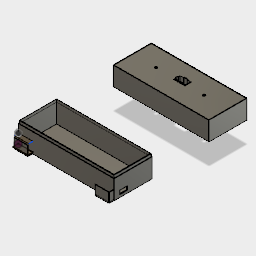
Breadboard case v11 (Autodesk Fusion 360 design; units mm, degrees)
Autodesk Fusion 360 part; units mm, degrees
sketch "Sketch1" plane through (0, 0, 0) normal (0, 1, 0) x (1, 0, 0)
  line L0 (100, 40) -> (-100, 40)
  line L1 (-100, 40) -> (-100, -40)
  line L2 (-100, -40) -> (100, -40)
  line L3 (100, -40) -> (100, 40)
  line L4 (100, 40) -> (-100, -40) construction
  line L5 (-100, 40) -> (100, -40) construction
  line L6 (-99, -39) -> (99, -39)
  line L7 (99, -39) -> (99, 39)
  line L8 (99, 39) -> (-99, 39)
  line L9 (-99, 39) -> (-99, -39)
  dimension "d1" = 200
  dimension "d2" = 80
  dimension "d3" = 1
  measures "d1" distance of L1.end L2.end
  measures "d2" distance of L0.end L1.end
extrude "Extrude1" add sketch "Sketch1" along normal blind 80 contours L0 L1 L2 L3 | L6 L7 L8 L9 makes body 1
shell "Shell1" thickness 1 removed faces 0 bodies 1
ref_plane "WorkPlane1" through (0, 40, 0) normal (0, 1, 0) x (0, 0, 1)
split "Split1" by plane through (0, 40, 0) normal (0, 1, 0) bodies 1 makes body 2 at (-33.3333, 80, -13.3333)
move_body "Move1" bodies 1 to x (1, 0, 0) y (0, 1, 0) z (0, 0, 1) at (-36.228, -3.4098, 161.9901)
sketch "Sketch2" plane through (0, -2.4098, 0) normal (0, 1, 0) x (-1, 0, 0)
  line L0 (-62.772, 200.9901) -> (-62.772, 122.9901)
  line L1 (-62.772, 122.9901) -> (135.228, 122.9901)
  line L2 (135.228, 122.9901) -> (135.228, 200.9901)
  line L3 (135.228, 200.9901) -> (-62.772, 200.9901)
  line L4 (135.228, 200.9901) -> (-62.772, 200.9901)
  line L5 (-62.772, 200.9901) -> (-62.772, 122.9901)
  line L6 (-62.772, 122.9901) -> (135.228, 122.9901)
  line L7 (135.228, 122.9901) -> (135.228, 200.9901)
  line L8 (-63.772, 121.9901) -> (136.228, 121.9901)
  line L9 (136.228, 121.9901) -> (136.228, 201.9901)
  line L10 (136.228, 201.9901) -> (-63.772, 201.9901)
  line L11 (-63.772, 201.9901) -> (-63.772, 121.9901)
  line L12 (135.228, 122.9901) -> (-62.772, 122.9901)
  line L13 (-62.772, 122.9901) -> (-62.772, 200.9901)
  line L14 (-62.772, 200.9901) -> (135.228, 200.9901)
  line L15 (135.228, 200.9901) -> (135.228, 122.9901)
  line L16 (-61.772, 199.9901) -> (-61.772, 123.9901)
  line L17 (-61.772, 123.9901) -> (134.228, 123.9901)
  line L18 (134.228, 123.9901) -> (134.228, 199.9901)
  line L19 (134.228, 199.9901) -> (-61.772, 199.9901)
  dimension "d7" = 1
  dimension "d8" = 1
extrude "Extrude2" add sketch "Sketch2" along normal blind 45 contours L0 L1 L2 L3 L4 L5 L6 L7 L12 L13 L14 L15 bodies 1
sketch "Sketch3" plane through (63.772, 0, 0) normal (1, 0, 0) x (0, 0, -1)
  line L0 (-121.9901, 36.5902) -> (-201.9901, 36.5902)
  line L1 (-201.9901, 36.5902) -> (-201.9901, -3.4098)
  line L2 (-201.9901, -3.4098) -> (-121.9901, -3.4098)
  line L3 (-121.9901, -3.4098) -> (-121.9901, 36.5902)
  line L4 (-190, 10) -> (-174, 10)
  line L5 (-174, 10) -> (-174, 2)
  line L6 (-174, 2) -> (-190, 2)
  line L7 (-190, 2) -> (-190, 10)
  dimension "d11" = 16
  dimension "d12" = 8
  measures "d11" distance of L4.start L4.end
  measures "d12" distance of L4.start L6.end
extrude "Extrude3" cut sketch "Sketch3" against normal up to surface (2 mm away) contours L4 L5 L6 L7 bodies 1
fillet "Fillet1" radius 0.5 4 edges at (-136.228, 16.5902, 121.9901) (-136.228, 16.5902, 201.9901) (63.772, 16.5902, 201.9901) (63.772, 16.5902, 121.9901) on bodies 1
chamfer "Chamfer1" distance 0.5 angle 45 4 edges at (-36.228, 42.5902, 200.9901) (62.772, 42.5902, 161.9901) (-36.228, 42.5902, 122.9901) (-135.228, 42.5902, 161.9901) on bodies 1
fillet "Fillet2" radius 0.5 9 edges at (0, 80, 40) (100, 80, 0) (100, 60, 40) (100, 60, -40) (0, 80, -40) (0, 40, -40) (-100, 80, 0) (-100, 40, 0) (0, 40, 40) on bodies 2
fillet "Fillet3" radius 0.5 9 edges at (-99.8536, 40.1464, -39.8536) (-100, 60, -40) (-99.8536, 79.8536, -39.8536) (-99.8536, 40.1464, 39.8536) (-100, 60, 40) (-99.8536, 79.8536, 39.8536) (-99, 79, 0) (0, 79, -39) (0, 79, 39) on bodies 2
sketch "Sketch4" plane through (0, 0, 121.9901) normal (0, 0, -1) x (-1, 0, 0)
  line L0 (-63.272, 36.5902) -> (-63.272, -3.4098)
  line L1 (-63.272, -3.4098) -> (135.728, -3.4098)
  line L2 (135.728, -3.4098) -> (135.728, 36.5902)
  line L3 (135.728, 36.5902) -> (-63.272, 36.5902)
  line L4 (-56, 18) -> (-40, 18)
  line L5 (-40, 18) -> (-40, 10)
  line L6 (-40, 10) -> (-56, 10)
  line L7 (-56, 10) -> (-56, 18)
  dimension "d19" = 16
  dimension "d20" = 8
  measures "d19" distance of L4.start L4.end
  measures "d20" distance of L4.start L6.end
extrude "Extrude4" cut sketch "Sketch4" against normal up to surface (4 mm away) contours L4 L5 L6 L7 bodies 1
sketch "Sketch7" plane through (0, 80, 0) normal (0, 1, 0) x (-1, 0, 0)
  arc A0 (-99.0001, 39.5) -> (-99.5, 39.0001) centre (-99.0001, 39.0001) ccw
  line L0 (-99.5, 39.0001) -> (-99.5, -39.0001)
  arc A1 (-99.5, -39.0001) -> (-99.0001, -39.5) centre (-99.0001, -39.0001) ccw
  line L1 (-99.0001, -39.5) -> (99.5, -39.5)
  line L2 (99.5, -39.5) -> (99.5, 39.5)
  line L3 (99.5, 39.5) -> (-99.0001, 39.5)
  line L4 (10, -10) -> (-12, -10)
  line L5 (-12, -10) -> (-12, 2)
  line L6 (-12, 2) -> (10, 2)
  line L7 (10, 2) -> (10, -10)
  dimension "d26" = 22
  dimension "d27" = 12
  measures "d26" distance of L4.start L4.end
  measures "d27" distance of L4.start L6.end
extrude "Extrude5" cut sketch "Sketch7" against normal up to surface (3 mm away) contours L4 L5 L6 L7 bodies 2
sketch "Sketch8" plane through (0, 80, 0) normal (0, 1, 0) x (-1, 0, 0)
  line L0 (10, 2) -> (10, -10)
  line L1 (10, -10) -> (-12, -10)
  line L2 (-12, -10) -> (-12, 2)
  line L3 (-12, 2) -> (10, 2)
  arc A0 (-99.0001, 39.5) -> (-99.5, 39.0001) centre (-99.0001, 39.0001) ccw
  line L4 (-99.5, 39.0001) -> (-99.5, -39.0001)
  arc A1 (-99.5, -39.0001) -> (-99.0001, -39.5) centre (-99.0001, -39.0001) ccw
  line L5 (-99.0001, -39.5) -> (99.5, -39.5)
  line L6 (99.5, -39.5) -> (99.5, 39.5)
  line L7 (99.5, 39.5) -> (-99.0001, 39.5)
  line L8 (11, -11) -> (-13, -11)
  line L9 (-13, -11) -> (-13, 3)
  line L10 (-13, 3) -> (11, 3)
  line L11 (11, 3) -> (11, -11)
  line L12 (-12, 2) -> (10, 2)
  line L13 (10, 2) -> (10, -10)
  line L14 (10, -10) -> (-12, -10)
  line L15 (-12, -10) -> (-12, 2)
  dimension "d30" = 1
extrude "Extrude6" add sketch "Sketch8" against normal blind 10 contours L8 L9 L10 L11 bodies 2
sketch "Sketch9" plane through (0, 80, 0) normal (0, 1, 0) x (-1, 0, 0)
  line L0 (10, 2) -> (10, -10)
  line L1 (10, -10) -> (-12, -10)
  line L2 (-12, -10) -> (-12, 2)
  line L3 (-12, 2) -> (10, 2)
  arc A0 (-99.0001, 39.5) -> (-99.5, 39.0001) centre (-99.0001, 39.0001) ccw
  line L4 (-99.5, 39.0001) -> (-99.5, -39.0001)
  arc A1 (-99.5, -39.0001) -> (-99.0001, -39.5) centre (-99.0001, -39.0001) ccw
  line L5 (-99.0001, -39.5) -> (99.5, -39.5)
  line L6 (99.5, -39.5) -> (99.5, 39.5)
  line L7 (99.5, 39.5) -> (-99.0001, 39.5)
  line L8 (12, -7) -> (10, -7)
  line L9 (10, -7) -> (10, -2)
  line L10 (10, -2) -> (12, -2)
  line L11 (12, -2) -> (12, -7)
  dimension "d33" = 5
  measures "d33" distance of L8.start L10.end
extrude "Extrude7" cut sketch "Sketch9" against normal blind 10 contours L0 L8 L9 L10 L11 bodies 2
sketch "Sketch10" plane through (0, 80, 0) normal (0, 1, 0) x (-1, 0, 0)
  line L0 (12, -7) -> (10, -7)
  line L1 (10, -7) -> (10, -10)
  line L2 (10, -10) -> (-12, -10)
  line L3 (-12, -10) -> (-12, 2)
  line L4 (-12, 2) -> (10, 2)
  line L5 (10, 2) -> (10, -2)
  line L6 (10, -2) -> (12, -2)
  line L7 (12, -2) -> (12, -7)
  arc A0 (-99.0001, 39.5) -> (-99.5, 39.0001) centre (-99.0001, 39.0001) ccw
  line L8 (-99.5, 39.0001) -> (-99.5, -39.0001)
  arc A1 (-99.5, -39.0001) -> (-99.0001, -39.5) centre (-99.0001, -39.0001) ccw
  line L9 (-99.0001, -39.5) -> (99.5, -39.5)
  line L10 (99.5, -39.5) -> (99.5, 39.5)
  line L11 (99.5, 39.5) -> (-99.0001, 39.5)
  line L12 (3, -12) -> (-5, -12)
  line L13 (-5, -12) -> (-5, -10)
  line L14 (-5, -10) -> (3, -10)
  line L15 (3, -10) -> (3, -12)
  dimension "d36" = 8
  measures "d36" distance of L12.start L12.end
extrude "Extrude8" cut sketch "Sketch10" against normal blind 20 contours L2 L12 L13 L14 L15 bodies 2
sketch "Sketch11" plane through (0, 80, 0) normal (0, 1, 0) x (-1, 0, 0)
  line L0 (-5, -12) -> (-5, -10)
  line L1 (-5, -10) -> (-12, -10)
  line L2 (-12, -10) -> (-12, 2)
  line L3 (-12, 2) -> (10, 2)
  line L4 (10, 2) -> (10, -2)
  line L5 (10, -2) -> (12, -2)
  line L6 (12, -2) -> (12, -7)
  line L7 (12, -7) -> (10, -7)
  line L8 (10, -7) -> (10, -10)
  line L9 (10, -10) -> (3, -10)
  line L10 (3, -10) -> (3, -12)
  line L11 (3, -12) -> (-5, -12)
  arc A0 (-99.0001, 39.5) -> (-99.5, 39.0001) centre (-99.0001, 39.0001) ccw
  line L12 (-99.5, 39.0001) -> (-99.5, -39.0001)
  arc A1 (-99.5, -39.0001) -> (-99.0001, -39.5) centre (-99.0001, -39.0001) ccw
  line L13 (-99.0001, -39.5) -> (99.5, -39.5)
  line L14 (99.5, -39.5) -> (99.5, 39.5)
  line L15 (99.5, 39.5) -> (-99.0001, 39.5)
  circle A2 centre (50, 0) radius 2.5
  dimension "d39" = 5
  measures "d39" diameter of A2
extrude "Extrude9" cut sketch "Sketch11" against normal blind 1 contours A2 bodies 2
sketch "Sketch12" plane through (0, 80, 0) normal (0, 1, 0) x (-1, 0, 0)
  circle A0 centre (50, 0) radius 2.5
  line L0 (-5, -12) -> (-5, -10)
  line L1 (-5, -10) -> (-12, -10)
  line L2 (-12, -10) -> (-12, 2)
  line L3 (-12, 2) -> (10, 2)
  line L4 (10, 2) -> (10, -2)
  line L5 (10, -2) -> (12, -2)
  line L6 (12, -2) -> (12, -7)
  line L7 (12, -7) -> (10, -7)
  line L8 (10, -7) -> (10, -10)
  line L9 (10, -10) -> (3, -10)
  line L10 (3, -10) -> (3, -12)
  line L11 (3, -12) -> (-5, -12)
  arc A1 (-99.0001, 39.5) -> (-99.5, 39.0001) centre (-99.0001, 39.0001) ccw
  line L12 (-99.5, 39.0001) -> (-99.5, -39.0001)
  arc A2 (-99.5, -39.0001) -> (-99.0001, -39.5) centre (-99.0001, -39.0001) ccw
  line L13 (-99.0001, -39.5) -> (99.5, -39.5)
  line L14 (99.5, -39.5) -> (99.5, 39.5)
  line L15 (99.5, 39.5) -> (-99.0001, 39.5)
  circle A3 centre (-50, 0) radius 2.5
  dimension "d42" = 5
  measures "d42" diameter of A3
extrude "Extrude10" cut sketch "Sketch12" against normal blind 1 contours A3 bodies 2
move_body "Move2" bodies 1 to x (1, 0, 0) y (0, 1, 0) z (0, 0, 1) at (0, 3, 0)
sketch "Sketch13" plane through (0, 0, 0) normal (0, 1, 0) x (1, 0, 0)
  line L0 (-135.728, -201.9901) -> (-105.728, -201.9901)
  line L1 (-105.728, -201.9901) -> (-105.728, -211.9901)
  line L2 (-105.728, -211.9901) -> (-135.728, -211.9901)
  line L3 (-135.728, -211.9901) -> (-135.728, -201.9901)
  line L4 (-136.728, -200.9901) -> (-104.728, -200.9901)
  line L5 (-104.728, -200.9901) -> (-104.728, -212.9901)
  line L6 (-104.728, -212.9901) -> (-136.728, -212.9901)
  line L7 (-136.728, -212.9901) -> (-136.728, -200.9901)
  point P0 (-135.728, -201.9901)
  dimension "d48" = 30
  dimension "d49" = 10
  dimension "d50" = 1
  measures "d48" distance of P0 L0.end
  measures "d49" distance of P0 L2.end
box "BoxPrimitive1" add length 10 width 30 height 20 placed x (0, 0, 1) y (1, 0, 0) z (0, 1, 0) at (-136, 0, 202) separate body makes body 3
sketch "Sketch15" plane through (0, 20, 0) normal (0, 1, 0) x (-1, 0, 0)
  line L0 (136, 212) -> (106, 212)
  line L1 (106, 212) -> (106, 202)
  line L2 (106, 202) -> (136, 202)
  line L3 (136, 202) -> (136, 212)
  line L4 (135, 202) -> (105, 202)
  line L5 (105, 202) -> (105, 211)
  line L6 (105, 211) -> (135, 211)
  line L7 (135, 211) -> (135, 202)
  dimension "d56" = 9
  dimension "d57" = 30
  measures "d56" distance of L4.start L6.end
  measures "d57" distance of L4.start L4.end
extrude "Extrude11" cut sketch "Sketch15" against normal blind 18 contours L1 L2 L4 L6 L7 | L1 L4 L5 L6 bodies 3
fillet "Fillet4" radius 1 2 edges at (-136, 10, 212) (-106, 10, 212) on bodies 3
copy_body "CopyPasteBodies1" bodies 3 makes body 4
move_body "Move3" bodies 4 to x (1, 0, 0) y (0, 1, 0) z (0, 0, 1) at (53.716, -13.548, 6.4975)
ref_plane "WorkPlane2" through (-67.284, -3.548, 212.9975) normal (-1, 0, 0) x (0, -1, 0)
mirror "Mirror1" about plane through (-67.284, -3.548, 212.9975) normal (-1, 0, 0) of bodies 4 makes body 5
move_body "Move4" bodies 5 to x (1, 0, 0) y (0, 1, 0) z (0, 0, 1) at (0, 0, 10)
move_body "Move5" bodies 5 to x (1, 0, 0) y (0, 1, 0) z (0, 0, 1) at (100, 0, 0)
move_body "Align1" bodies 5 to x (1, 0, 0) y (0, 1, 0) z (0, 0, 1) at (15.556, 0, -17.0074)
move_body "Align2" bodies 1 to x (1, 0, 0) y (0, 1, 0) z (0, 0, 1) at (0, -13.1382, -0.5)
move_body "Align3" bodies 4 to x (1, 0, 0) y (0, 1, 0) z (0, 0, 1) at (0, 0, -10.2229)
move_body "Move6" bodies 4 to x (1, 0, 0) y (0, 1, 0) z (0, 0, 1) at (0, 0, 100)
move_body "Align4" bodies 3 to x (1, 0, 0) y (0, 1, 0) z (0, 0, 1) at (0, -13.548, -0.5099)
move_body "Move7" bodies 3 5 1 to x (1, 0, 0) y (0, 1, 0) z (0, 0, 1) at (0, 10, 0)
hidden bodies 4
